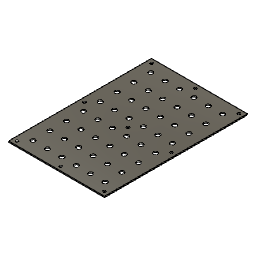
Kapton v2 (Autodesk Fusion 360 design; units mm, degrees)
Autodesk Fusion 360 part; units mm, degrees
sketch "Sketch1" plane through (0, 0, 0) normal (0, 0, 1) x (1, 0, 0)
  line L0 (42.595, 63.475) -> (-42.595, 63.475)
  line L1 (-42.595, 63.475) -> (-42.595, -63.475)
  line L2 (-42.595, -63.475) -> (42.595, -63.475)
  line L3 (42.595, -63.475) -> (42.595, 63.475)
  line L4 (42.595, 63.475) -> (-42.595, -63.475) construction
  line L5 (-42.595, 63.475) -> (42.595, -63.475) construction
  line L6 (37.095, 57.275) -> (-37.095, 57.275)
  line L7 (-37.095, 57.275) -> (-37.095, -57.275)
  line L8 (-37.095, -57.275) -> (37.095, -57.275)
  line L9 (37.095, -57.275) -> (37.095, 57.275)
  line L10 (37.095, 57.275) -> (-37.095, -57.275) construction
  line L11 (-37.095, 57.275) -> (37.095, -57.275) construction
  line L12 (34.095, 54.275) -> (-34.095, 54.275)
  line L13 (-34.095, 54.275) -> (-34.095, -54.275)
  line L14 (-34.095, -54.275) -> (34.095, -54.275)
  line L15 (34.095, -54.275) -> (34.095, 54.275)
  line L16 (34.095, 54.275) -> (-34.095, -54.275) construction
  line L17 (-34.095, 54.275) -> (34.095, -54.275) construction
  dimension "d1" = 85.19
  dimension "d2" = 126.95
  dimension "d3" = 74.19
  dimension "d4" = 114.55
  dimension "d5" = 68.19
  dimension "d6" = 108.55
  constraint horizontal L0
  constraint perpendicular L0 L1
  constraint parallel L0 L2
  constraint parallel L1 L3
  constraint coincident L4 origin
  constraint coincident L5 origin
  constraint horizontal L6
  constraint perpendicular L6 L7
  constraint parallel L6 L8
  constraint parallel L7 L9
  constraint coincident L10 origin
  constraint coincident L11 origin
  constraint horizontal L12
  constraint perpendicular L12 L13
  constraint parallel L12 L14
  constraint parallel L13 L15
  constraint coincident L16 origin
  constraint coincident L17 origin
  measures "d1" distance of L1.end L2.end
  measures "d2" distance of L0.end L1.end
  measures "d3" distance of L7.end L8.end
  measures "d4" distance of L6.end L7.end
  measures "d5" distance of L13.end L14.end
  measures "d6" distance of L12 L14
sketch "Sketch2" plane through (0, 0, 0) normal (0, 0, 1) x (1, 0, 0)
sketch "Sketch3" plane through (0, 0, 0) normal (0, 0, 1) x (1, 0, 0)
  line L0 (34.095, 54.275) -> (-34.095, 54.275)
  line L1 (-34.095, 54.275) -> (-34.095, -54.275)
  circle A0 centre (-32.095, 52.275) radius 2
  dimension "d7" = 2
  constraint tangent L0 A0
  constraint tangent L1 A0
  measures "d7" radius of A0
extrude "Extrude1" add sketch "Sketch1" along normal blind 1 contours L0 L1 L2 L3 | L6 L7 L8 L9 | L12 L13 L14 L15
sketch "Sketch4" plane through (0, 0, 0) normal (0, 0, 1) x (1, 0, 0)
sketch "Sketch5" plane through (0, 0, 1) normal (0, 0, 1) x (-1, 0, 0)
  line L0 (-42.595, 63.475) -> (-42.595, -63.475)
  line L1 (-42.595, -63.475) -> (42.595, -63.475)
  line L2 (42.595, -63.475) -> (42.595, 63.475)
  line L3 (42.595, 63.475) -> (-42.595, 63.475)
  line L4 (-34.095, 54.275) -> (34.095, 54.275)
  line L5 (34.095, 54.275) -> (34.095, -54.275)
  line L6 (34.095, -54.275) -> (-34.095, -54.275)
  line L7 (-34.095, -54.275) -> (-34.095, 54.275)
  line L8 (-34.095, 54.275) -> (34.095, -54.275) construction
  line L9 (34.095, 54.275) -> (-34.095, -54.275) construction
  circle A0 centre (32.095, -52.275) radius 2
  dimension "d10" = 68.19
  dimension "d11" = 108.55
  dimension "d12" = 2
  constraint horizontal L4
  constraint perpendicular L4 L5
  constraint parallel L4 L6
  constraint parallel L5 L7
  constraint coincident L8 origin
  constraint coincident L9 origin
  constraint tangent L5 A0
  constraint tangent L6 A0
  measures "d10" distance of L5.end L6.end
  measures "d11" distance of L4.end L5.end
  measures "d12" radius of A0
loft "Loft1" cut profiles "Sketch5", "Sketch3" section 1 contours A0 section 2 contours A0
pattern_linear "R-Pattern1" count 6 spacing 12.8 along (1, 0, 0) count 8 spacing 14.9286 along (0, -1, 0) of "Loft1"
sketch "Sketch6" plane through (0, 0, 1) normal (0, 0, 1) x (-1, 0, 0)
  circle A0 centre (0, 0) radius 1.5
  circle A1 centre (0, -59.81) radius 1.5
  circle A2 centre (0, 59.81) radius 1.5
  circle A3 centre (38.77, -59.81) radius 1.5
  circle A4 centre (38.77, 0) radius 1.5
  circle A5 centre (38.77, 59.81) radius 1.5
  circle A6 centre (-38.77, 0) radius 1.5
  circle A7 centre (-38.77, 59.81) radius 1.5
  circle A8 centre (-38.77, -59.81) radius 1.5
  dimension "d17" = 3
  dimension "d18" = 59.81
  dimension "d19" = 3
  dimension "d20" = 59.81
  dimension "d21" = 3
  dimension "d23" = 3
  dimension "d24" = 3
  dimension "d25" = 59.81
  dimension "d26" = 3
  dimension "d28" = 3
  dimension "d29" = 3
  dimension "d30" = 59.81
  dimension "d31" = 3
  constraint coincident A0.centre origin
  measures "d17" diameter of A0
  measures "d18" distance of A0.centre A1.centre
  measures "d19" diameter of A1
  measures "d20" distance of A0.centre A2.centre
  measures "d21" diameter of A2
  measures "d23" diameter of A4
  measures "d24" diameter of A3
  measures "d25" distance of A4.centre A5.centre
  measures "d26" diameter of A5
  measures "d28" diameter of A6
  measures "d29" diameter of A8
  measures "d30" distance of A6.centre A7.centre
  measures "d31" diameter of A7
hole "Hole1" at (-38.77, 59.81, 1) at (0, 59.81, 1) at (38.77, 59.81, 1) at (38.77, 0, 1) at (-38.77, 0, 1) at (-38.77, -59.81, 1) at (0, -59.81, 1) at (38.77, -59.81, 1) at (0, 0, 1) direction (0, 0, -1) diameter 2.529 depth 14 tip angle 180
thread "Thread1" "ISO Metric profile 3.0 M3x0.5 6H" thread offset 0 thread depth 7.4
